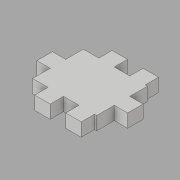
# Autodesk Inventor part: g_arm 2
Saved by Autodesk Inventor 2019 (Build 230136000, 136)
## iProperties
Created: 2021-11-01
Part Number: g_arm 2
Material: Generic
Document SubType Name: Modeling
Designer: Mohamed
Density: 1 g/cm^3
Appearance: Default
Author: Mohamed
Autodesk Inventor part; units mm, degrees
ref_plane "YZ Plane" through (0, 0, 0) normal (1, 0, 0) x (0, 1, 0)
ref_plane "XZ Plane" through (0, 0, 0) normal (0, 1, 0) x (-1, 0, 0)
ref_plane "XY Plane" through (0, 0, 0) normal (0, 0, 1) x (1, 0, 0)
sketch "Sketch1" plane through (0, 0, 0) normal (0, 1, 0) x (-1, 0, 0)
  line L0 (0, 0) -> (35, 0)
  line L1 (35, 0) -> (35, -21)
  line L2 (35, -21) -> (0, -21)
  line L3 (0, -21) -> (0, 0)
  dimension "d0" = 35
  dimension "d1" = 21
  constraints: 8 end point, 2 parallel, 1 horizontal, 1 perpendicular
  measures "d0" distance of L1.end L2.end
  measures "d1" distance of L0.end L1.end
extrude "Extrusion1" add sketch "Sketch1" along normal blind 6
sketch "Sketch2" plane through (0, 6, 0) normal (0, 1, 0) x (1, 0, 0)
  line L0 (-35, 21) -> (-35, 0) projected
  line L1 (-35, 0) -> (-29, 0)
  line L2 (-29, 0) -> (-29, 7)
  line L3 (-29, 7) -> (-35, 7)
  line L4 (-35, 7) -> (-35, 0)
  point P0 (0, 0)
  dimension "d4" = 6
  dimension "d5" = 7
  constraints: 8 end point, 2 parallel, 1 horizontal, 1 perpendicular
  measures "d4" distance of L3.end L2.end
  measures "d5" distance of L2.end L1.end
extrude "Extrusion2" cut sketch "Sketch2" against normal blind 6
pattern_linear "Rectangular Pattern1" count 2 spacing 14 along (0, 0, -1) of "Extrusion2"
sketch "Sketch3" plane through (0, 6, 0) normal (0, 1, 0) x (1, 0, 0)
  line L0 (-29, 7) -> (-29, 0) projected
  line L1 (-29, 0) -> (0, 0)
  line L2 (0, 0) -> (0, -1)
  line L3 (0, -1) -> (-29, -1)
  line L4 (-29, -1) -> (-29, 0)
  line L5 (-29, 14) -> (-29, 21) projected
  line L6 (-29, 21) -> (0, 21)
  line L7 (0, 21) -> (0, 22)
  line L8 (0, 22) -> (-29, 22)
  line L9 (-29, 22) -> (-29, 21)
  point P0 (0, 0)
  dimension "d11" = 29
  dimension "d12" = 1
  dimension "d13" = 29
  dimension "d14" = 1
  constraints: 16 end point, 4 parallel, 2 horizontal, 2 perpendicular
  measures "d11" distance of L2.end L3.end
  measures "d12" distance of L1.end L2.end
  measures "d13" distance of L8.end L7.end
  measures "d14" distance of L7.end L6.end
extrude "Extrusion3" add sketch "Sketch3" against normal blind 6
sketch "Sketch4" plane through (0, 6, 0) normal (0, 1, 0) x (1, 0, 0)
  line L0 (-29, -1) -> (-29, 7) projected
  line L1 (0, 22) -> (0, -1) projected
  line L2 (0, 7) -> (6, 7)
  line L3 (6, 7) -> (6, 14)
  line L4 (6, 14) -> (0, 14)
  line L5 (0, 14) -> (0, 7)
  point P0 (0, 0)
  dimension "d17" = 6
  dimension "d18" = 7
  constraints: 8 end point, 2 parallel, 1 horizontal, 1 perpendicular, 1 point on line
  measures "d17" distance of L4.end L3.end
  measures "d18" distance of L3.end L2.end
extrude "Extrusion4" add sketch "Sketch4" against normal blind 6
sketch "Sketch5" plane through (0, 6, 0) normal (0, 1, 0) x (1, 0, 0)
  line L0 (0, -1) -> (-29, -1) projected
  line L1 (-29, -1) -> (-22, -1)
  line L2 (-22, -1) -> (-22, -7)
  line L3 (-22, -7) -> (-15, -7)
  line L4 (-15, -7) -> (-15, -1)
  line L5 (-29, 22) -> (0, 22) projected
  line L6 (-29, 22) -> (-22, 22)
  line L7 (-22, 22) -> (-22, 28)
  line L8 (-22, 28) -> (-15, 28)
  line L9 (-15, 28) -> (-15, 22)
  point P0 (0, 0)
  dimension "d22" = 6
  dimension "d23" = 7
  dimension "d25" = 6
  dimension "d26" = 7
  constraints: 16 end point, 6 perpendicular, 4 point on line
  measures "d22" distance of L1.end L2.end
  measures "d23" distance of L2.end L3.end
  measures "d25" distance of L6.end L7.end
  measures "d26" distance of L7.end L8.end
extrude "Extrusion5" add sketch "Sketch5" against normal blind 6
pattern_linear "Rectangular Pattern2" count 2 spacing 14 along (1, 0, 0) of "Extrusion5"
body "Solid1"
